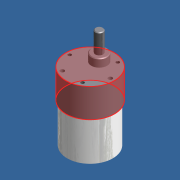
# Autodesk Inventor part: conrad_getriebe_motor
Saved by Autodesk Inventor 2014 SP2 (Build 180246200, 246)
## iProperties
Created: 2012-05-08
Part Number: conrad_getriebe_motor
Material: Stahl
Document SubType Name: Modeling
Designer: 4ndreas
Mass: 417.146 g
Surface Area: 106.462 cm^2
Volume: 53.1397 cm^3
Density: 7.85 g/cm^3
Appearance: Stahl
Author: 4ndreas
Autodesk Inventor part; units mm, degrees
ref_plane "YZ Plane" through (0, 0, 0) normal (1, 0, 0) x (0, 1, 0)
ref_plane "XZ Plane" through (0, 0, 0) normal (0, 1, 0) x (-1, 0, 0)
ref_plane "XY Plane" through (0, 0, 0) normal (0, 0, 1) x (1, 0, 0)
sketch "Skizze1" plane through (0, 0, 0) normal (0, 0, 1) x (1, 0, 0)
  circle A0 centre (7.75, -13.4234) radius 1.5
  circle A1 centre (-7.75, -13.4234) radius 1.5
  circle A2 centre (-13.4234, 7.75) radius 1.5
  circle A3 centre (13.4234, 7.75) radius 1.5
  circle A4 centre (-7.75, 13.4234) radius 1.5
  circle A5 centre (15.5, 0) radius 1.5
  circle A6 centre (7.75, 13.4234) radius 1.5
  circle A7 centre (0, -15.5) radius 1.5
  circle A8 centre (-15.5, 0) radius 1.5
  circle A9 centre (0, 7) radius 6
  circle A10 centre (0, 0) radius 18.5
  constraints: 11 centre point, 23 other
extrude "Extrusion1" add sketch "Skizze1" along normal blind 6 contours A9
extrude "Extrusion2" add sketch "Skizze1" against normal blind 22 contours A0 | A1 | A2 | A3 | A4 | A5 | A6 | A7 | A8 | A9 | A10
sketch "Skizze2" plane through (0, 0, -22) normal (0, 0, -1) x (-1, 0, 0)
  circle A0 centre (0, 0) radius 18.5 projected
  circle A1 centre (0, 0) radius 17.4
  dimension "d4" = 34.8
  constraints: 1 centre point, 1 coincident
  measures "d4" diameter of A1
extrude "Extrusion3" add sketch "Skizze2" along normal blind 30 separate body contours A1
chamfer "Fase1" distance 0.5 angle 45 1 edges at (-6, 7, 6)
sketch "Skizze3" plane through (0, 7, 6) normal (0, 0, 1) x (1, 0, 0)
  circle A0 centre (0, 0) radius 5.5 projected
  circle A1 centre (0, 0) radius 3
  point P0 (0, -7)
  dimension "d10" = 6
  constraints: 1 centre point, 1 coincident
  measures "d10" diameter of A1
extrude "Extrusion4" add sketch "Skizze3" along normal blind 15 separate body contours A1
chamfer "Fase2" distance 0.5 angle 45 1 edges at (-3, 7, 21)
extrude "Extrusion5" cut sketch "Skizze1" against normal blind 4 contours A1 | A4 | A5 bodies 1
hole "Bohrung1" at (-15.5, 0, 0) at (7.75, -13.4234, 0) at (7.75, 13.4234, 0) direction (0, 0, -1) diameter 2.459 depth 4 tip angle 118 bodies 1 thread size "M3x0.5" class "6H" standard "ANSI Metric M Profile"
sketch "Skizze4" plane through (0, 7, 21) normal (0, 0, 1) x (1, 0, 0)
  circle A0 centre (0, 0) radius 2.5 projected
  circle A1 centre (0, 0) radius 3 projected
  line L0 (-1.6583, 2.5) -> (1.6583, 2.5)
  point P0 (0, -7)
  dimension "d25" = 5.5
  constraints: 2 end point, 2 point on circle
extrude "Extrusion6" cut sketch "Skizze4" against normal blind 12 contours L0 A1 picked at (-0.897, 2.6056) bodies 3
